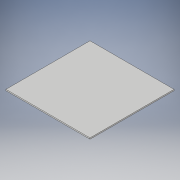
# Autodesk Inventor part: Top Plate
Saved by Autodesk Inventor 2019 (Build 230136000, 136)
## iProperties
Created: 2019-03-05
Part Number: Top Plate
Material: Nylon 6/6
Document SubType Name: Modeling
Designer: Delta
Density: 1.13 g/cm^3
Appearance: Default
Mass: 1417.74 g
Surface Area: 4064.51 cm^2
Volume: 1254.63 cm^3
Author: Delta
Autodesk Inventor part; units mm, degrees
ref_plane "YZ Plane" through (0, 0, 0) normal (1, 0, 0) x (0, 1, 0)
ref_plane "XZ Plane" through (0, 0, 0) normal (0, 1, 0) x (-1, 0, 0)
ref_plane "XY Plane" through (0, 0, 0) normal (0, 0, 1) x (1, 0, 0)
sketch "Sketch1" plane through (0, 0, 0) normal (0, 1, 0) x (-1, 0, 0)
  line L0 (0, 0) -> (444.5, 0)
  line L1 (444.5, 0) -> (444.5, -444.5)
  line L2 (444.5, -444.5) -> (0, -444.5)
  line L3 (0, -444.5) -> (0, 0)
  dimension "d0" = 444.5
  dimension "d1" = 444.5
  constraints: 8 end point, 2 parallel, 1 horizontal, 1 perpendicular
  measures "d0" distance of L1.end L2.end
  measures "d1" distance of L0.end L1.end
extrude "Extrusion1" add sketch "Sketch1" along normal blind 6.35
body "Solid1"
